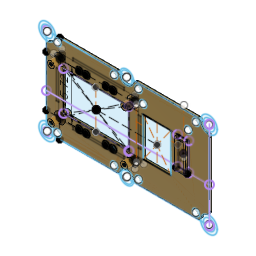
Proto Insert v14 v1 v14 (Autodesk Fusion 360 design; units mm, degrees)
Autodesk Fusion 360 part; units mm, degrees
sketch "Sketch1" plane through (0, 0, 0) normal (0, 1, 0) x (1, 0, 0) in component "Proto Board Adapter"
  circle A0 centre (71.7181, 0.0098) radius 6.2
  circle A1 centre (60.5472, -3.6571) radius 3
  circle A2 centre (71.7181, 0.0098) radius 2
  circle A3 centre (60.5448, -74.3595) radius 1.25
  circle A4 centre (60.5472, -3.6571) radius 1.25
  line L0 (146.4189, -78.6553) -> (-0.6746, -78.6553)
  circle A5 centre (9.5469, -74.3657) radius 3
  circle A6 centre (9.5469, -74.3657) radius 1.25
  circle A7 centre (86.7325, -64.7668) radius 3
  circle A8 centre (146.0095, -0.0026) radius 7.4
  circle A9 centre (134.2864, -74.3595) radius 3
  circle A10 centre (134.2989, -3.6579) radius 1.25
  circle A11 centre (-0.0163, -78.0309) radius 5
  circle A12 centre (145.9932, -78.0335) radius 7.4
  circle A13 centre (134.2989, -3.6579) radius 3
  circle A14 centre (9.5493, -3.6633) radius 3
  circle A15 centre (82.55, -3.654) radius 1.25
  line L1 (146.4189, 0.8132) -> (146.4189, -78.6553)
  circle A16 centre (0, 0) radius 5
  circle A17 centre (146.0095, -0.0026) radius 2
  circle A18 centre (86.7325, -64.7668) radius 1.25
  circle A19 centre (0, 0) radius 7.4
  circle A20 centre (-0.0163, -78.0309) radius 7.4
  circle A21 centre (82.5375, -74.3556) radius 1.25
  circle A22 centre (82.55, -3.654) radius 3
  circle A23 centre (9.5493, -3.6633) radius 1.25
  circle A24 centre (145.9932, -78.0335) radius 2
  circle A25 centre (127.4333, -64.7704) radius 3
  circle A26 centre (127.4333, -64.7704) radius 1.25
  circle A27 centre (-0.0163, -78.0309) radius 2
  circle A28 centre (82.5375, -74.3556) radius 3
  circle A29 centre (146.0095, -0.0026) radius 5
  line L2 (-0.6746, -78.6553) -> (-0.6746, 0.8132)
  circle A30 centre (0, 0) radius 2
  circle A31 centre (145.9932, -78.0335) radius 5
  line L3 (-0.6746, 0.8132) -> (146.4189, 0.8132)
  circle A32 centre (71.7181, 0.0098) radius 5
  circle A33 centre (71.7181, -78.04) radius 6.2
  circle A34 centre (134.2864, -74.3595) radius 1.25
  circle A35 centre (71.7181, -78.04) radius 2
  circle A36 centre (60.5448, -74.3595) radius 3
  circle A37 centre (71.7181, -78.04) radius 5
  point P0 (72.1438, -78.6618)
  point P1 (72.1439, -0.612)
  dimension "d12" = 2.5
  dimension "d13" = 6
  dimension "d14" = 2.5
  dimension "d15" = 6
  dimension "d16" = 2.5
  dimension "d17" = 6
  dimension "d18" = 2.5
  dimension "d19" = 6
  dimension "d20" = 2.5
  dimension "d21" = 6
  dimension "d22" = 2.5
  dimension "d23" = 6
  dimension "d24" = 2.5
  dimension "d25" = 6
  dimension "d26" = 2.5
  dimension "d27" = 6
  dimension "d28" = 2.5
  dimension "d29" = 6
  dimension "d30" = 2.5
  dimension "d31" = 6
  dimension "d32" = 4
  dimension "d33" = 10
  dimension "d34" = 4
  dimension "d35" = 10
  dimension "d36" = 4
  dimension "d37" = 10
  dimension "d38" = 4
  dimension "d39" = 10
  dimension "d40" = 4
  dimension "d41" = 10
  dimension "d42" = 4
  dimension "d43" = 10
  dimension "d120" = 147.0934
  dimension "d121" = 79.4685
  constraint concentric A25 A26
  constraint concentric A9 A34
  constraint concentric A7 A18
  constraint concentric A21 A28
  constraint concentric A3 A36
  constraint concentric A5 A6
  constraint concentric A1 A4
  constraint concentric A14 A23
  constraint concentric A10 A13
  constraint concentric A15 A22
  constraint concentric A24 A31
  constraint concentric A17 A29
  constraint concentric A11 A27
  constraint concentric A16 A30
  constraint horizontal L0
  constraint vertical L2
  constraint horizontal L3
  constraint vertical L1
  constraint concentric A35 A37
  constraint concentric A2 A32
  measures "d12" diameter of A26
  measures "d13" diameter of A25
  measures "d14" diameter of A34
  measures "d15" diameter of A9
  measures "d16" diameter of A18
  measures "d17" diameter of A7
  measures "d18" diameter of A21
  measures "d19" diameter of A28
  measures "d20" diameter of A3
  measures "d21" diameter of A36
  measures "d22" diameter of A6
  measures "d23" diameter of A5
  measures "d24" diameter of A4
  measures "d25" diameter of A1
  measures "d26" diameter of A23
  measures "d27" diameter of A14
  measures "d28" diameter of A10
  measures "d29" diameter of A13
  measures "d30" diameter of A15
  measures "d31" diameter of A22
  measures "d32" diameter of A24
  measures "d33" diameter of A31
  measures "d34" diameter of A17
  measures "d35" diameter of A29
  measures "d36" diameter of A27
  measures "d37" diameter of A11
  measures "d38" diameter of A30
  measures "d39" diameter of A16
  measures "d40" diameter of A35
  measures "d41" diameter of A37
  measures "d42" diameter of A2
  measures "d43" diameter of A32
  measures "d120" distance of L1 L2
  measures "d121" distance of L0 L3
sketch "Sketch2" plane through (0, 0, 0) normal (0, 1, 0) x (1, 0, 0) in component "Proto Board Adapter"
  circle A0 centre (77.3654, -61.7811) radius 3
  circle A1 centre (35.4554, -16.0611) radius 1.25
  circle A2 centre (29.1054, -61.7811) radius 1.25
  circle A3 centre (59.5854, -16.0611) radius 3
  circle A4 centre (77.3654, -61.7811) radius 1.25
  circle A5 centre (53.2354, -61.7811) radius 1.25
  circle A6 centre (35.4554, -61.7811) radius 1.25
  circle A7 centre (35.4554, -61.7811) radius 3
  circle A8 centre (53.2354, -61.7811) radius 3
  circle A9 centre (53.2354, -16.0611) radius 1.25
  circle A10 centre (29.1054, -16.0611) radius 3
  circle A11 centre (53.2354, -16.0611) radius 3
  circle A12 centre (59.5854, -16.0611) radius 1.25
  circle A13 centre (29.1054, -61.7811) radius 3
  circle A14 centre (59.5854, -61.7811) radius 3
  circle A15 centre (11.3254, -61.7811) radius 3
  circle A16 centre (59.5854, -61.7811) radius 1.25
  circle A17 centre (11.3254, -16.0611) radius 3
  circle A18 centre (77.3654, -16.0611) radius 1.25
  circle A19 centre (11.3254, -16.0611) radius 1.25
  circle A20 centre (11.3254, -61.7811) radius 1.25
  circle A21 centre (29.1054, -16.0611) radius 1.25
  circle A22 centre (35.4554, -16.0611) radius 3
  circle A23 centre (77.3654, -16.0611) radius 3
  line L0 (11.3254, -61.7811) -> (11.3254, -78.6553) construction
  line L1 (11.3254, -16.0611) -> (11.3254, 0.8132) construction
  line L2 (-0.6746, 0.8132) -> (146.4189, 0.8132) construction
  line L3 (146.4189, -78.6553) -> (-0.6746, -78.6553) construction
  line L4 (11.3254, -61.7811) -> (29.1054, -61.7811) construction
  line L5 (29.1054, -61.7811) -> (35.4554, -61.7811) construction
  line L6 (35.4554, -61.7811) -> (53.2354, -61.7811) construction
  line L7 (53.2354, -61.7811) -> (59.5854, -61.7811) construction
  line L8 (59.5854, -61.7811) -> (77.3654, -61.7811) construction
  line L9 (11.3254, -61.7811) -> (-0.6746, -61.7811) construction
  line L10 (-0.6746, -78.6553) -> (-0.6746, 0.8132) construction
  line L11 (11.3254, -61.7811) -> (77.3654, -16.0611) construction
  line L12 (77.3654, -61.7811) -> (11.3254, -16.0611) construction
  line L13 (11.3254, -16.0611) -> (-0.6746, -16.0611) construction
  point P0 (44.3454, -38.9211)
  dimension "d44" = 2.5
  dimension "d45" = 6
  dimension "d46" = 2.5
  dimension "d47" = 6
  dimension "d50" = 2.5
  dimension "d51" = 6
  dimension "d53" = 6
  dimension "d54" = 2.5
  dimension "d55" = 6
  dimension "d56" = 2.5
  dimension "d57" = 6
  dimension "d58" = 2.5
  dimension "d59" = 6
  dimension "d60" = 2.5
  dimension "d61" = 6
  dimension "d70" = 2.5
  dimension "d71" = 6
  dimension "d72" = 2.5
  dimension "d73" = 6
  dimension "d74" = 2.5
  dimension "d75" = 6
  dimension "d76" = 2.5
  dimension "d77" = 6
  dimension "d97" = 45.72
  dimension "d98" = 45.72
  dimension "d99" = 45.72
  dimension "d100" = 45.72
  dimension "d101" = 45.72
  dimension "d102" = 45.72
  dimension "d107" = 17.78
  dimension "d108" = 17.78
  dimension "d109" = 17.78
  dimension "d110" = 17.78
  dimension "d111" = 6.35
  dimension "d112" = 6.35
  dimension "d113" = 6.35
  dimension "d115" = 6.35
  dimension "d116" = 17.78
  dimension "d117" = 17.78
  dimension "d124" = 12
  constraint concentric A0 A4
  constraint concentric A18 A23
  constraint concentric A14 A16
  constraint concentric A3 A12
  constraint concentric A5 A8
  constraint concentric A9 A11
  constraint concentric A6 A7
  constraint concentric A1 A22
  constraint concentric A2 A13
  constraint concentric A10 A21
  constraint concentric A15 A20
  constraint concentric A17 A19
  constraint coincident A15.centre A20.centre
  constraint vertical L0
  constraint coincident A17.centre A19.centre
  constraint vertical L1
  constraint coincident L1.end L2
  constraint coincident L0.end L3
  constraint equal L0 L1
  constraint coincident A2.centre A13.centre
  constraint horizontal L4
  constraint coincident A6.centre A7.centre
  constraint coincident A5.centre A8.centre
  constraint horizontal L6
  constraint coincident A14.centre A16.centre
  constraint parallel L6 L7
  constraint coincident A0.centre A4.centre
  constraint parallel L7 L8
  constraint horizontal L5
  constraint perpendicular L0 L9
  constraint coincident L9.end L10
  constraint coincident A18.centre A23.centre
  constraint midpoint L11 P0
  constraint coincident L10 L13.end
  constraint perpendicular L10 L13
  constraint equal L9 L13
  measures "d44" diameter of A4
  measures "d45" diameter of A0
  measures "d46" diameter of A18
  measures "d47" diameter of A23
  measures "d50" diameter of A16
  measures "d51" diameter of A14
  measures "d53" diameter of A3
  measures "d54" diameter of A5
  measures "d55" diameter of A8
  measures "d56" diameter of A9
  measures "d57" diameter of A11
  measures "d58" diameter of A6
  measures "d59" diameter of A7
  measures "d60" diameter of A1
  measures "d61" diameter of A22
  measures "d70" diameter of A2
  measures "d71" diameter of A13
  measures "d72" diameter of A21
  measures "d73" diameter of A10
  measures "d74" diameter of A20
  measures "d75" diameter of A15
  measures "d76" diameter of A19
  measures "d77" diameter of A17
  measures "d97" distance of A0.centre A18.centre
  measures "d98" distance of A3.centre A14.centre
  measures "d99" vertical distance of A9.centre A5.centre
  measures "d100" vertical distance of A1.centre A6.centre
  measures "d101" vertical distance of A2.centre A10.centre
  measures "d102" vertical distance of A15.centre A17.centre
  measures "d107" distance of A0.centre A14.centre
  measures "d108" distance of A18.centre A3.centre
  measures "d109" distance of A5.centre A6.centre
  measures "d110" distance of A9.centre A1.centre
  measures "d111" distance of A5.centre A14.centre
  measures "d112" distance of A3.centre A9.centre
  measures "d113" distance of A1.centre A10.centre
  measures "d115" distance of A6.centre A2.centre
  measures "d116" distance of A15.centre A2.centre
  measures "d117" distance of A10.centre A17.centre
  measures "d124" distance of A15.centre L9.end
sketch "Sketch3" plane through (0, 0, 0) normal (0, 1, 0) x (1, 0, 0) in component "Proto Board Adapter"
  line L0 (73.8454, -56.4211) -> (73.8454, -21.4211)
  line L1 (14.8454, -21.4211) -> (14.8454, -56.4211)
  line L2 (14.8454, -56.4211) -> (73.8454, -56.4211)
  line L3 (73.8454, -21.4211) -> (14.8454, -21.4211)
  line L4 (73.8454, -56.4211) -> (14.8454, -21.4211) construction
  line L5 (14.8454, -56.4211) -> (73.8454, -21.4211) construction
  point P0 (44.3454, -38.9211)
  point P1 (44.3454, -38.9211)
  dimension "d154" = 59
  dimension "d155" = 35
  constraint horizontal L2
  constraint vertical L0
  constraint horizontal L3
  constraint vertical L1
  constraint midpoint L4 P1
  constraint coincident P1 P0
  measures "d154" distance of L1.end L0.start
  measures "d155" distance of L1.start L1.end
sketch "Sketch4" plane through (0, 0, 0) normal (0, 1, 0) x (1, 0, 0) in component "Proto Board Adapter"
  line L0 (117.8454, -56.4211) -> (127.8454, -56.4211)
  line L1 (127.8454, -56.4211) -> (127.8454, -31.4211)
  line L2 (127.8454, -31.4211) -> (117.8454, -31.4211)
  line L3 (117.8454, -31.4211) -> (117.8454, -56.4211)
  line L4 (118.8454, -56.4211) -> (126.8454, -56.4211)
  line L5 (126.8454, -56.4211) -> (126.8454, -31.4211)
  line L6 (126.8454, -31.4211) -> (118.8454, -31.4211)
  line L7 (118.8454, -31.4211) -> (118.8454, -56.4211)
  line L8 (117.8454, -56.4211) -> (127.8454, -31.4211) construction
  line L9 (127.8454, -56.4211) -> (117.8454, -31.4211) construction
  line L10 (118.8454, -56.4211) -> (126.8454, -31.4211) construction
  line L11 (126.8454, -56.4211) -> (118.8454, -31.4211) construction
  line L12 (73.8454, -56.4211) -> (73.8454, -21.4211) construction
  line L13 (73.8454, -56.4211) -> (117.8454, -56.4211) construction
  point P0 (122.8454, -43.9211)
  point P1 (122.8454, -43.9211)
  point P2 (44.3454, -38.9211)
  dimension "d126" = 10
  dimension "d128" = 8
  dimension "d129" = 25
  dimension "d191" = 44
  constraint horizontal L0
  constraint vertical L1
  constraint horizontal L2
  constraint vertical L3
  constraint horizontal L4
  constraint vertical L5
  constraint horizontal L6
  constraint vertical L7
  constraint coincident L0 L4.start
  constraint midpoint L11 P1
  constraint midpoint L8 P1
  constraint coincident P1 P0
  constraint coincident L12.start L13.start
  constraint horizontal L13
  measures "d126" distance of L0.start L0.end
  measures "d128" distance of L4.start L4.end
  measures "d129" distance of L4.start L6.end
  measures "d191" distance of L3 L12
sketch "Sketch5" plane through (0, 0, 0) normal (0, 1, 0) x (1, 0, 0) in component "Proto Board Adapter"
  line L0 (111.6706, -56.4211) -> (86.6706, -56.4211)
  line L1 (86.6706, -56.4211) -> (86.6706, -21.4211)
  line L2 (86.6706, -21.4211) -> (111.6706, -21.4211)
  line L3 (111.6706, -21.4211) -> (111.6706, -56.4211)
  line L4 (146.4189, 0.8132) -> (146.4189, -78.6553)
  line L5 (127.8454, -56.4211) -> (127.8454, -31.4211)
  line L6 (86.6706, -56.4211) -> (111.6706, -21.4211) construction
  line L7 (111.6706, -56.4211) -> (86.6706, -21.4211) construction
  line L8 (99.1706, -38.9211) -> (44.3454, -38.9211) construction
  line L9 (123.3822, -41.1005) -> (123.3822, -81.8799) construction
  line L10 (80.4959, -61.6286) -> (80.4959, -16.4077) construction
  line L11 (80.4959, -47.6613) -> (86.6706, -47.6613) construction
  line L12 (111.6706, -48.2742) -> (117.8454, -48.2742) construction
  line L13 (117.8454, -31.4211) -> (117.8454, -56.4211) construction
  line L14 (99.1706, -56.4211) -> (99.1706, -21.4211) construction
  line L15 (43.9261, -56.4211) -> (43.9261, -21.4211) construction
  line L16 (14.8454, -56.4211) -> (73.8454, -56.4211) construction
  line L17 (73.8454, -21.4211) -> (14.8454, -21.4211) construction
  point P0 (99.1706, -38.9211)
  point P1 (122.8454, -43.9211)
  point P2 (44.3454, -38.9211)
  dimension "d133" = 25
  constraint horizontal L0
  constraint vertical L1
  constraint horizontal L2
  constraint vertical L3
  constraint midpoint L6 P0
  constraint coincident P0 L8.start
  constraint horizontal L8
  constraint coincident P2 L8.end
  constraint perpendicular L0 L9
  constraint parallel L5 L10
  constraint coincident L10 L11.start
  constraint coincident L1 L11.end
  constraint perpendicular L1 L11
  constraint coincident L3 L12.start
  constraint perpendicular L3 L12
  constraint equal L11 L12
  constraint coincident L12.end L13
  constraint midpoint L0 L14.start
  constraint midpoint L2 L14.end
  constraint vertical L15
  constraint coincident L15.start L16
  constraint coincident L15.end L17
  constraint equal L14 L15
  measures "d133" distance of L0.start L0.end
extrude "Extrude1" add sketch "Sketch1" along normal blind 2 contours A0 L0 A5 A8 A12 A14 L1 A19 A20 L2 L3 A33 | A14 A19 | A5 A20 | A1 | A7 | A9 | A13 | A18 | A22 | A25 | A26 | A28 | A36 picked at (7.2201, -3.3347) picked at (7.3767, -75.1677) in component "Proto Board Adapter"
extrude "Extrude2" add sketch "Sketch2" along normal blind 8 contours A0 | A4 | A15 | A17 | A18 | A19 | A20 | A23 in component "Proto Board Adapter"
extrude "Extrude3" add sketch "Sketch2" against normal blind 8 contours A0 | A4 | A15 | A17 | A18 | A19 | A20 | A23 in component "Proto Board Adapter"
hole "Hole1" at (11.3254, -8, 61.7811) direction (0, 1, 0) diameter 2.175 depth 6 tip angle 180 in component "Proto Board Adapter"
thread "Thread1" "ISO Metric profile 2.6 M2.6x0.45 6H" major diameter 2.675 minor diameter 2.1754 pitch 0.45 angle 60 modelled right hand crest width 0.1241 on face at (10.4425, -6, 61.1462) crest through (11.3254, -7.8875, 60.6934) in component "Proto Board Adapter"
hole "Hole2" at (77.3654, -8, 61.7811) direction (0, 1, 0) diameter 2.175 depth 6 tip angle 180 in component "Proto Board Adapter"
thread "Thread2" "ISO Metric profile 2.6 M2.6x0.45 6H" major diameter 2.675 minor diameter 2.1754 pitch 0.45 angle 60 modelled right hand crest width 0.1241 on face at (76.943, -6, 60.779) crest through (77.3654, -7.8875, 60.6934) in component "Proto Board Adapter"
hole "Hole3" at (77.3654, -8, 16.0611) direction (0, 1, 0) diameter 2.175 depth 6 tip angle 180 in component "Proto Board Adapter"
thread "Thread3" "ISO Metric profile 2.6 M2.6x0.45 6H" major diameter 2.675 minor diameter 2.1754 pitch 0.45 angle 60 modelled right hand crest width 0.1241 on face at (76.943, -6, 15.059) crest through (77.3654, -7.8875, 14.9734) in component "Proto Board Adapter"
hole "Hole4" at (11.3254, -8, 16.0611) direction (0, 1, 0) diameter 2.175 depth 6 tip angle 180 in component "Proto Board Adapter"
thread "Thread4" "ISO Metric profile 2.6 M2.6x0.45 6H" major diameter 2.675 minor diameter 2.1754 pitch 0.45 angle 60 modelled right hand crest width 0.1241 on face at (11.3797, -6, 14.9749) crest through (11.3254, -7.8875, 14.9734) in component "Proto Board Adapter"
extrude "Extrude5" add sketch "Sketch4" against normal blind 4 in component "Proto Board Adapter"
sketch "Sketch6" plane through (0, 0, 31.4211) normal (0, 0, -1) x (1, 0, 0) in component "Proto Board Adapter"
  line L0 (117.8454, 0) -> (127.8454, 0)
  line L1 (127.8454, 0) -> (127.8454, 4)
  line L2 (127.8454, 4) -> (117.8454, 4)
  line L3 (117.8454, 4) -> (117.8454, 0)
  line L4 (126.8454, 0) -> (118.8454, 0)
  line L5 (118.8454, 0) -> (118.8454, 3)
  line L6 (118.8454, 3) -> (126.8454, 3)
  line L7 (126.8454, 3) -> (126.8454, 0)
  line L8 (-0.6746, 0) -> (146.4189, 0)
  line L9 (117.8454, 1.5) -> (118.8454, 1.5) construction
  line L10 (126.8454, 1.5) -> (127.8454, 1.5) construction
  dimension "d159" = 8
  dimension "d160" = 3
  constraint horizontal L4
  constraint vertical L5
  constraint horizontal L6
  constraint vertical L7
  constraint coincident L0 L4.start
  constraint coincident L3 L9.start
  constraint midpoint L5 L9.end
  constraint midpoint L7 L10.start
  constraint coincident L1 L10.end
  constraint perpendicular L1 L10
  constraint horizontal L9
  constraint equal L9 L10
  measures "d159" distance of L5 L7
  measures "d160" distance of L6 L8
extrude "Extrude6" cut sketch "Sketch6" against normal up to surface (25 mm away) contours L0 L4 L5 L6 L7 L8 in component "Proto Board Adapter"
fillet "Fillet1" radius 3 12 edges at (138.6193, 1, 78.6553) (146.4189, 1, 70.6458) (65.5487, 1, 78.6553) (77.8875, 1, 78.6553) (7.3573, 1, 78.6553) (-0.6746, 1, 70.6602) (-0.6746, 1, 7.3692) (7.3552, 1, -0.8132) (77.8659, 1, -0.8132) (65.5704, 1, -0.8132) (138.6546, 1, -0.8132) (146.4189, 1, 7.3913) in component "Proto Board Adapter"
fillet "Fillet3" radius 1 6 edges at (127.8454, 0, 43.9211) (127.8454, -4, 43.9211) (117.8454, 0, 43.9211) (117.8454, -4, 43.9211) (126.8454, -3, 43.9211) (118.8454, -3, 43.9211) in component "Proto Board Adapter"
fillet "Fillet4" radius 2 4 edges at (74.5685, 0, 62.8659) (8.5285, 0, 62.8659) (8.5285, 0, 17.1459) (74.5685, 0, 17.1459) in component "Proto Board Adapter"
sketch "Sketch7" plane through (0, 2, 0) normal (0, 1, 0) x (-1, 0, 0) in component "Proto Board Adapter"
  arc A0 (-146.4189, 10.0748) -> (-144.1662, 7.1693) centre (-143.4189, 10.0748) ccw
  arc A1 (-138.7745, 1.5568) -> (-144.1662, 7.1693) centre (-146.0095, 0.0026) ccw
  arc A2 (-138.7745, 1.5568) -> (-135.8415, -0.8132) centre (-135.8415, 2.1868) ccw
  line L0 (-135.8415, -0.8132) -> (-80.6521, -0.8132)
  arc A3 (-80.6521, -0.8132) -> (-77.7388, 1.4705) centre (-80.6521, 2.1868) ccw
  arc A4 (-65.6975, 1.4705) -> (-77.7388, 1.4705) centre (-71.7181, -0.0098) ccw
  arc A5 (-65.6975, 1.4705) -> (-62.7842, -0.8132) centre (-62.7842, 2.1868) ccw
  line L1 (-62.7842, -0.8132) -> (-10.1675, -0.8132)
  arc A6 (-10.1675, -0.8132) -> (-7.2346, 1.556) centre (-10.1675, 2.1868) ccw
  arc A7 (-1.6546, 7.2126) -> (-7.2346, 1.556) centre (0, 0) ccw
  arc A8 (-1.6546, 7.2126) -> (0.6746, 10.1367) centre (-2.3254, 10.1367) ccw
  line L2 (0.6746, 10.1367) -> (0.6746, 67.898)
  arc A9 (0.6746, 67.898) -> (-1.6499, 70.8209) centre (-2.3254, 67.898) ccw
  arc A10 (-7.188, 76.3406) -> (-1.6499, 70.8209) centre (0.0163, 78.0309) ccw
  arc A11 (-7.188, 76.3406) -> (-10.1087, 78.6553) centre (-10.1087, 75.6553) ccw
  line L3 (-10.1087, 78.6553) -> (-62.8325, 78.6553)
  arc A12 (-62.8325, 78.6553) -> (-65.73, 76.4329) centre (-62.8325, 75.6553) ccw
  arc A13 (-77.7062, 76.4329) -> (-65.73, 76.4329) centre (-71.7181, 78.04) ccw
  arc A14 (-77.7062, 76.4329) -> (-80.6037, 78.6553) centre (-80.6037, 75.6553) ccw
  line L4 (-80.6037, 78.6553) -> (-135.8687, 78.6553)
  arc A15 (-135.8687, 78.6553) -> (-138.7892, 76.3413) centre (-135.8687, 75.6553) ccw
  arc A16 (-144.1615, 70.8638) -> (-138.7892, 76.3413) centre (-145.9932, 78.0335) ccw
  arc A17 (-144.1615, 70.8638) -> (-146.4189, 67.9571) centre (-143.4189, 67.9571) ccw
  line L5 (-146.4189, 67.9571) -> (-146.4189, 10.0748)
  circle A18 centre (-11.3254, 16.0611) radius 3
  circle A19 centre (-11.3254, 61.7811) radius 3
  circle A20 centre (-77.3654, 16.0611) radius 3
  circle A21 centre (-77.3654, 61.7811) radius 3
  circle A22 centre (-9.5469, 74.3657) radius 1.25
  circle A23 centre (-60.5448, 74.3595) radius 1.25
  circle A24 centre (-134.2989, 3.6579) radius 1.25
  circle A25 centre (-82.55, 3.654) radius 1.25
  circle A26 centre (-9.5493, 3.6633) radius 1.25
  circle A27 centre (-82.5375, 74.3556) radius 1.25
  circle A28 centre (-60.5472, 3.6571) radius 1.25
  circle A29 centre (-134.2864, 74.3595) radius 1.25
  line L6 (-67.3654, 66.7811) -> (-21.3254, 66.7811)
  line L7 (-21.3254, 66.7811) -> (-21.3254, 64.7811)
  line L8 (-21.3254, 64.7811) -> (-67.3654, 64.7811)
  line L9 (-67.3654, 64.7811) -> (-67.3654, 66.7811)
  line L10 (-21.3254, 11.0611) -> (-67.3654, 11.0611)
  line L11 (-67.3654, 11.0611) -> (-67.3654, 13.0611)
  line L12 (-67.3654, 13.0611) -> (-21.3254, 13.0611)
  line L13 (-21.3254, 13.0611) -> (-21.3254, 11.0611)
  line L14 (-82.3654, 51.7811) -> (-80.3654, 51.7811)
  line L15 (-80.3654, 51.7811) -> (-80.3654, 26.0611)
  line L16 (-80.3654, 26.0611) -> (-82.3654, 26.0611)
  line L17 (-82.3654, 26.0611) -> (-82.3654, 51.7811)
  line L18 (-8.3254, 26.0611) -> (-8.3254, 51.7811)
  line L19 (-8.3254, 51.7811) -> (-6.3254, 51.7811)
  line L20 (-6.3254, 51.7811) -> (-6.3254, 26.0611)
  line L21 (-6.3254, 26.0611) -> (-8.3254, 26.0611)
  line L22 (-77.3654, 61.7811) -> (-77.3654, 66.1919) construction
  line L23 (-67.3654, 64.7811) -> (-77.3654, 64.7811) construction
  line L24 (-11.3254, 61.7811) -> (-11.3254, 69.0928) construction
  line L25 (-21.3254, 64.7811) -> (-11.3254, 64.7811) construction
  line L26 (-77.3654, 61.7811) -> (-82.7529, 61.7811) construction
  line L27 (-11.3254, 61.7811) -> (-3.9006, 61.7811) construction
  line L28 (-8.3254, 51.7811) -> (-8.3254, 61.7811) construction
  line L29 (-77.3654, 16.0611) -> (-85.3306, 16.0611) construction
  line L30 (-80.3654, 26.0611) -> (-80.3654, 16.0611) construction
  line L31 (-80.3654, 51.7811) -> (-80.3654, 61.7811) construction
  line L32 (-8.3254, 26.0611) -> (-8.3254, 16.0611) construction
  line L33 (-77.3654, 16.0611) -> (-77.3654, 8.3417) construction
  line L34 (-67.3654, 13.0611) -> (-77.3654, 13.0611) construction
  line L35 (-21.3254, 13.0611) -> (-11.3254, 13.0611) construction
  dimension "d178" = 2
  dimension "d179" = 2
  dimension "d180" = 2
  dimension "d181" = 2
  dimension "d184" = 10
  dimension "d185" = 10
  dimension "d186" = 10
  dimension "d187" = 10
  constraint horizontal L6
  constraint vertical L7
  constraint horizontal L8
  constraint vertical L9
  constraint horizontal L12
  constraint vertical L13
  constraint horizontal L10
  constraint vertical L11
  constraint horizontal L14
  constraint vertical L15
  constraint horizontal L16
  constraint vertical L17
  constraint horizontal L19
  constraint vertical L20
  constraint horizontal L21
  constraint vertical L18
  constraint coincident A21.centre L22.start
  constraint vertical L22
  constraint coincident L22 L23.end
  constraint coincident A21 L23.end
  constraint coincident A19.centre L24.start
  constraint coincident L24 L25.end
  constraint coincident A19 L25.end
  constraint horizontal L25
  constraint equal L23 L25
  constraint perpendicular L22 L26
  constraint perpendicular L24 L27
  constraint coincident L27 L28.end
  constraint coincident A19 L28.end
  constraint vertical L28
  constraint coincident A20.centre L29.start
  constraint perpendicular L15 L29
  constraint coincident L29 L30.end
  constraint coincident A20 L30.end
  constraint coincident L26 L31.end
  constraint coincident A21 L31.end
  constraint vertical L31
  constraint vertical L30
  constraint coincident A18 L32.end
  constraint tangent A18 L32
  constraint perpendicular L21 L32
  constraint equal L30 L31
  constraint equal L28 L32
  constraint perpendicular L29 L33
  constraint coincident L33 L34.end
  constraint coincident A20 L34.end
  constraint coincident A18 L35.end
  constraint horizontal L34
  constraint horizontal L35
  constraint equal L34 L35
  measures "d178" distance of L6.start L8.end
  measures "d179" distance of L11.end L10.end
  measures "d180" distance of L15 L17
  measures "d181" distance of L18 L20
  measures "d184" distance of L18.end L28.end
  measures "d185" distance of L7.end L25.end
  measures "d186" distance of L14.end L31.end
  measures "d187" distance of L11.end L34.end
extrude "Extrude8" add sketch "Sketch7" along normal blind 4 contours L6 L7 L8 L9 | L10 L11 L12 L13 | L14 L15 L16 L17 | L18 L19 L20 L21 in component "Proto Board Adapter"
extrude "Extrude9" cut sketch "Sketch5" sketch "Sketch3" along normal blind 2 of sketch 2 in component "Proto Board Adapter"
fillet "Fillet5" radius 2 8 edges at (86.6706, 1, 21.4211) (86.6706, 1, 56.4211) (111.6706, 1, 56.4211) (111.6706, 1, 21.4211) (73.8454, 1, 21.4211) (73.8454, 1, 56.4211) (14.8454, 1, 21.4211) (14.8454, 1, 56.4211) in component "Proto Board Adapter"
component "Proto Board Adapter" placed x (1, 0, 0) y (0, 1, 0) z (0, 0, 1) at (0, 0, 0)
equation "d97 = ProtoWidth"
equation "d98 = ProtoWidth"
equation "d99 = ProtoWidth"
equation "d100 = ProtoWidth"
equation "d101 = ProtoWidth"
equation "d102 = ProtoWidth"
equation "d107 = ProtoGap"
equation "d108 = ProtoGap"
equation "d109 = ProtoGap"
equation "d110 = ProtoGap"
equation "d111 = ProtoHoleGap"
equation "d112 = ProtoHoleGap"
equation "d113 = ProtoHoleGap"
equation "d115 = ProtoHoleGap"
equation "d116 = ProtoGap"
equation "d117 = ProtoGap"
equation "d135 = MountingPlateThickness"
equation "d137 = StandoffBottomHeight + MountingPlateThickness"
equation "d139 = -StandoffTopHeight"
equation "d141 = StandoffHoleDepth"
equation "d144 = StandoffHoleDepth"
equation "d147 = StandoffHoleDepth"
equation "d150 = StandoffHoleDepth"
equation "d169 = SmallFillet"
equation "MountingPlateThickness = 2 mm"
equation "StandoffBottomHeight = 6 mm"
equation "StandoffHoleDepth = 6 mm"
equation "MountingPlateFillet = 2 mm"
equation "StandoffTopHeight = 8 mm"
equation "SmallFillet = 1 mm"
equation "d177 = MountingPlateFillet"
equation "d178 = MountingPlateThickness"
equation "d179 = MountingPlateThickness"
equation "d180 = MountingPlateThickness"
equation "d181 = MountingPlateThickness"
equation "BatteryHolderHeight = StandoffBottomHeight - 2 mm"
equation "d189 = BatteryHolderHeight"
equation "d192 = MountingPlateThickness"
equation "d195 = MountingPlateFillet"
